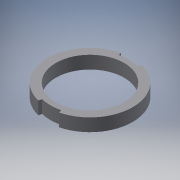
# Autodesk Inventor part: Battery Tube Collar
Saved by Autodesk Inventor 2016 (Build 200138000, 138)
## iProperties
Created: 2015-06-17
Part Number: Battery Tube Collar
Material: Generic
Document SubType Name: Modeling
Designer: JR
Density: 1 g/cm^3
Appearance: Default
Author: JR
Autodesk Inventor part; units mm, degrees
ref_plane "YZ Plane" through (0, 0, 0) normal (1, 0, 0) x (0, 1, 0)
ref_plane "XZ Plane" through (0, 0, 0) normal (0, 1, 0) x (-1, 0, 0)
ref_plane "XY Plane" through (0, 0, 0) normal (0, 0, 1) x (1, 0, 0)
sketch "Sketch1" plane through (0, 0, 0) normal (0, 0, 1) x (1, 0, 0)
  circle A0 centre (0, 0) radius 16
  circle A1 centre (0, 0) radius 20
  dimension "d0" = 32
  dimension "d1" = 40
  constraints: 2 centre point, 2 coincident
  measures "d0" diameter of A0
  measures "d1" diameter of A1
extrude "Extrusion1" add sketch "Sketch1" along normal blind 6
sketch "Sketch2" plane through (0, 0, 6) normal (0, 0, 1) x (1, 0, 0)
  line L0 (-4.3061, 18.5) -> (4.6939, 18.5) construction
  line L1 (-4.5, 20) -> (4.5, 20) construction
  circle A0 centre (0, 0) radius 20 construction
  circle A1 centre (0, 0) radius 20 projected
  arc A2 (4.8649, 19.3993) -> (-4.8649, 19.3993) centre (0, 0) ccw
  arc A3 (4.5, 17.9444) -> (-4.5, 17.9444) centre (0, 0) ccw
  line L2 (4.5, 17.9444) -> (4.8649, 19.3993)
  line L3 (-4.5, 17.9444) -> (-4.8649, 19.3993)
  line L4 (-4.8649, 19.3993) -> (0, 0) construction
  line L5 (4.8649, 19.3993) -> (0, 0) construction
  circle A4 centre (0, 0) radius 16 construction
  line L6 (-16, 0) -> (16, 0) construction
  arc A5 (-4.8649, -19.3993) -> (4.8649, -19.3993) centre (0, 0) ccw
  arc A6 (-4.5, -17.9444) -> (4.5, -17.9444) centre (0, 0) ccw
  line L7 (4.5, -17.9444) -> (4.8649, -19.3993)
  line L8 (-4.5, -17.9444) -> (-4.8649, -19.3993)
  point P0 (0, 20)
  point P1 (0, -20)
  dimension "d4" = 9
  dimension "d5" = 1.5
  constraints: 18 end point, 14 point on circle, 5 symmetric about line, 4 centre point, 3 horizontal, 3 vertical alignment, 2 collinear, 2 concentric, 2 tangent, 1 midpoint, 1 parallel, 2 other
  measures "d4" distance of L1.start L1.end
  measures "d5" distance between parallel lines of L0 L1
extrude "Extrusion2" cut sketch "Sketch2" against normal through all contours L2 A3 L3 A1 | A1 L8 A6 L7
equation "\"d1\" = BattECOD"
equation "\"d5\" = GripLength"
equation "\"BattECOD\" = 40"
equation "\"GripLength\" = 1.5"
body "Solid1"
